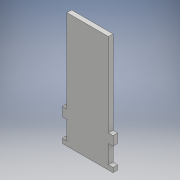
# Autodesk Inventor part: k2_t_l4-01
Saved by Autodesk Inventor 2017 (Build 210142000, 142)
## iProperties
Created: 2017-02-10
Part Number: k2_t_l4-01
Material: Generic
Document SubType Name: Modeling
Designer: herman
Density: 1 g/cm^3
Appearance: Default
d2: 3,000 mm
d3: 0,00 deg
d8: 3,000 mm
d9: 3,000 mm
d11: 33,000 mm
d12: 6,000 mm
d13: 60,415 mm
d14: 12,000 mm
Author: herman
Autodesk Inventor part; units mm, degrees
ref_plane "YZ Plane" through (0, 0, 0) normal (1, 0, 0) x (0, 1, 0)
ref_plane "XZ Plane" through (0, 0, 0) normal (0, 1, 0) x (-1, 0, 0)
ref_plane "XY Plane" through (0, 0, 0) normal (0, 0, 1) x (1, 0, 0)
sketch "Sketch1" plane through (0, 0, 0) normal (0, 1, 0) x (-1, 0, 0)
  line L0 (16.7962, 5.6332) -> (-10.2038, 5.6332)
  line L1 (-13.2038, -66.7819) -> (-13.2038, -69.7819)
  line L2 (-13.2038, -69.7819) -> (19.7962, -69.7819)
  line L3 (19.7962, -69.7819) -> (19.7962, -66.7819)
  line L4 (19.7962, -54.7819) -> (16.7962, -54.7819)
  line L5 (16.7962, -54.7819) -> (16.7962, -66.7819)
  line L6 (16.7962, -66.7819) -> (19.7962, -66.7819)
  line L7 (-13.2038, -66.7819) -> (-10.2038, -66.7819)
  line L8 (-10.2038, -66.7819) -> (-10.2038, -54.7819)
  line L9 (-10.2038, -54.7819) -> (-13.2038, -54.7819)
  line L10 (19.7962, -54.7819) -> (19.7962, -48.7819)
  line L11 (19.7962, -48.7819) -> (16.7962, -48.7819)
  line L12 (16.7962, -48.7819) -> (16.7962, 5.6332)
  line L13 (-13.2038, -54.7819) -> (-13.2038, -48.7819)
  line L14 (-13.2038, -48.7819) -> (-10.2038, -48.7819)
  line L15 (-10.2038, -48.7819) -> (-10.2038, 5.6332)
  dimension "d8" = 3
  dimension "d9" = 3
  dimension "d11" = 33
  dimension "d12" = 6
  dimension "d13" = 60.4152
  dimension "d14" = 12
  constraints: 32 end point, 10 perpendicular, 7 equal length, 2 horizontal, 2 point on line, 2 vertical, 1 parallel
  measures "d8" distance of L5.end L3.end
  measures "d9" distance of L2.end L3.end
  measures "d11" distance of L1.end L2.end
  measures "d12" distance of L4.start L10.end
  measures "d13" distance of L0.start L4.end
  measures "d14" distance of L4.end L5.end
extrude "Extrusion1" add sketch "Sketch1" along normal blind 3
body "Solid1"
